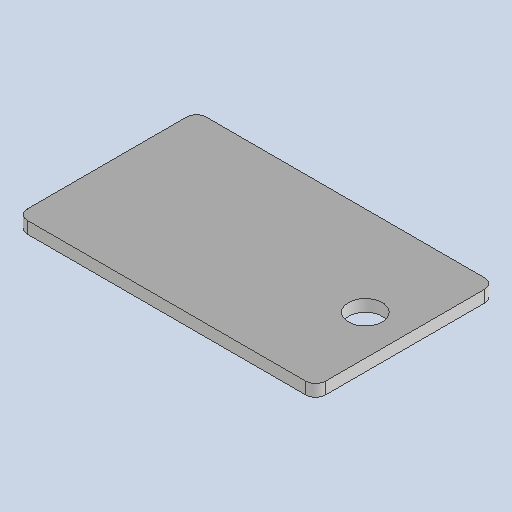
# Autodesk Inventor part: PRS 9695 leg floor plate_1200
Saved by Autodesk Inventor 2026.2 (Build 302298000, 298)
## iProperties
Created: 2025-02-20
Part Number: PRS 9695 leg floor plate_1200
Material: Stainless Steel
Document SubType Name: Sheet Metal
Designer: admin
Mass: 599.447 g
Surface Area: 281.235 cm^2
Volume: 74.9308 cm^3
Density: 8 g/cm^3
Flat Pattern Width: 9 cm
Flat Pattern Length: 15 cm
Flat Pattern Area: 135 cm^2
Sheet Metal Rule: AISI304 3mm Die 32
Sheet Metal Width: 90,000 mm
Sheet Metal Length: 150,000 mm
Sheet Metal Area: 13500,000 mm^2
Appearance: Default
Author: user
Autodesk Inventor part; units mm, degrees
ref_plane "YZ Plane" through (0, 0, 0) normal (1, 0, 0) x (0, 1, 0)
ref_plane "XZ Plane" through (0, 0, 0) normal (0, 1, 0) x (-1, 0, 0)
ref_plane "XY Plane" through (0, 0, 0) normal (0, 0, 1) x (1, 0, 0)
sketch "Sketch1" plane through (0, 0, 0) normal (0, 0, 1) x (1, 0, 0)
  line L0 (-75, -45) -> (75, -45)
  line L1 (75, -45) -> (75, 45)
  line L2 (75, 45) -> (-75, 45)
  line L3 (-75, 45) -> (-75, -45)
  line L4 (-75, -45) -> (75, 45) construction
  line L5 (75, -45) -> (-75, 45) construction
  circle A0 centre (55, -25) radius 8.5
  circle A1 centre (55, 25) radius 8.5
  line L6 (0, 0) -> (75, 0) construction
  circle A2 centre (55, 0) radius 8.5
  dimension "d0" = 150
  dimension "d1" = 90
  dimension "d23" = 17
  dimension "d25" = 20
  dimension "d26" = 20
  measures "d0" distance of L2.end L1.end
  measures "d1" distance of L1.end L0.end
  measures "d23" diameter of A0
  measures "d25" distance from line of L1 A0.centre
  measures "d26" distance from line of A0.centre L0
extrude "Plate1" add sketch "Sketch1" along normal blind 6 contours L3 L2 L1 L0 | A0 | A1
fillet "Corner Round2" radius 5 4 edges at (-75, 45, 3) (-75, -45, 3) (75, -45, 3) (75, 45, 3)
equation "\"d26\" = d25"
equation "\"d2\" = Thickness"
equation "\"BendReliefWidth\" = Thickness"
equation "\"BendReliefDepth\" = 0.5 * Thickness"
equation "\"CornerReliefSize\" = 4 * Thickness"
equation "\"MinimumRemnant\" = 2 * Thickness"
equation "\"TransitionRadius\" = BendRadius"
equation "\"JacobiRadiusSize\" = BendRadius"
equation "\"GapSize\" = Thickness"
equation "\"Thickness\" = 6"
equation "\"BendRadius\" = 5"
body "Solid1"
